Autodesk Fusion 360 part; units mm, degrees
note: some values were not read from the file. Set by a fixed rule: which sketch regions a step uses.
(part 3 of 4)
  spline S86 degree 3 poles (-105.7651, -158.0876) (-108.1851, -156.9591) (-106.086, -147.5724) (-100.1317, -132.8949) knots 0 0 0 0 1 1 1 1
  spline S87 degree 3 poles (-100.1317, -132.8949) (-98.7815, -129.5666) (-97.5292, -125.0086) (-97.3489, -122.7659) knots 0 0 0 0 1 1 1 1
  spline S88 degree 3 poles (-97.3489, -122.7659) (-97.1686, -120.5233) (-96.5325, -118.1966) (-95.9356, -117.5951) knots 0 0 0 0 1 1 1 1
  spline S89 degree 3 poles (-95.9356, -117.5951) (-95.3387, -116.9936) (-94.113, -114.2518) (-93.212, -111.5023) knots 0 0 0 0 1 1 1 1
  spline S90 degree 3 poles (-93.212, -111.5023) (-91.5685, -106.4875) (-88.2032, -100.9795) (-84.6693, -97.5197) knots 0 0 0 0 1 1 1 1
  spline S91 degree 3 poles (-84.6693, -97.5197) (-83.6282, -96.5006) (-82.5684, -95.831) (-82.3142, -96.0317) knots 0 0 0 0 1 1 1 1
  spline S92 degree 3 poles (-82.3142, -96.0317) (-80.8591, -97.1801) (-81.4531, -105.6318) (-83.0888, -107.0535) knots 0 0 0 0 1 1 1 1
  spline S93 degree 3 poles (-83.0888, -107.0535) (-83.9086, -107.766) (-83.3399, -110.3472) (-82.4356, -110.0181) knots 0 0 0 0 1 1 1 1
  spline S94 degree 3 poles (-82.4356, -110.0181) (-81.5449, -109.6939) (-77.0276, -113.218) (-76.5096, -114.6411) knots 0 0 0 0 1 1 1 1
  spline S95 degree 3 poles (-76.5096, -114.6411) (-76.1157, -115.7233) (-75.6688, -115.8539) (-74.1947, -115.3174) knots 0 0 0 0 1 1 1 1
  spline S96 degree 3 poles (-74.1947, -115.3174) (-73.0292, -114.8932) (-71.9308, -114.9941) (-71.1607, -115.5962) knots 0 0 0 0 1 1 1 1
  spline S97 degree 3 poles (-71.1607, -115.5962) (-70.4967, -116.1152) (-69.7314, -116.4591) (-69.4601, -116.3603) knots 0 0 0 0 1 1 1 1
  spline S98 degree 3 poles (-69.4601, -116.3603) (-69.1888, -116.2616) (-67.7713, -116.3006) (-66.31, -116.4471) knots 0 0 0 0 1 1 1 1
  spline S99 degree 3 poles (-66.31, -116.4471) (-58.7633, -116.1747) (-54.7735, -110.4959) (-53.9972, -105.1142) knots 0 0 0 0 1 1 1 1
  spline S100 degree 3 poles (-53.9972, -105.1142) (-53.3719, -100.2884) (-56.959, -94.4448) (-60.8927, -93.8814) knots 0 0 0 0 1 1 1 1
  spline S101 degree 3 poles (-60.8927, -93.8814) (-63.6579, -93.4851) (-63.887, -92.6055) (-62.4815, -87.7805) knots 0 0 0 0 1 1 1 1
  spline S102 degree 3 poles (-62.4815, -87.7805) (-60.4144, -80.6836) (-58.6819, -56.2234) (-59.8595, -50.7648) knots 0 0 0 0 1 1 1 1
  spline S103 degree 3 poles (-59.8595, -50.7648) (-60.45, -48.0282) (-60.4959, -47.9901) (-66.1098, -45.5661) knots 0 0 0 0 1 1 1 1
  spline S104 degree 3 poles (-66.1098, -45.5661) (-72.7999, -42.6775) (-79.68, -40.6969) (-84.3741, -40.3079) knots 0 0 0 0 1 1 1 1
  spline S105 degree 3 poles (-84.3741, -40.3079) (-87.8752, -40.018) (-88.8355, -39.1456) (-87.7319, -37.2577) knots 0 0 0 0 1 1 1 1
  spline S106 degree 3 poles (-87.7319, -37.2577) (-87.3803, -36.6562) (-87.2231, -35.8055) (-87.3826, -35.3672) knots 0 0 0 0 1 1 1 1
  spline S107 degree 3 poles (-87.3826, -35.3672) (-87.8899, -33.9734) (-86.4389, -25.012) (-85.4231, -23.2654) knots 0 0 0 0 1 1 1 1
  spline S108 degree 3 poles (-85.4231, -23.2654) (-84.2448, -21.2393) (-84.8036, -21.3276) (-87.2116, -23.5478) knots 0 0 0 0 1 1 1 1
  spline S109 degree 3 poles (-87.2116, -23.5478) (-88.988, -25.1857) (-89.0133, -25.1867) (-89.5753, -23.6426) knots 0 0 0 0 1 1 1 1
  spline S110 degree 3 poles (-89.5753, -23.6426) (-91.0986, -20.9242) (-96.5777, -20.042) (-99.4834, -22.2152) knots 0 0 0 0 1 1 1 1
  spline S111 degree 3 poles (-99.4834, -22.2152) (-102.7671, -24.1219) (-105.1902, -27.5695) (-103.4783, -30.4373) knots 0 0 0 0 1 1 1 1
  spline S112 degree 3 poles (-103.4783, -30.4373) (-102.821, -31.518) (-102.6423, -32.3115) (-103.0249, -32.4507) knots 0 0 0 0 1 1 1 1
  spline S113 degree 3 poles (-103.0249, -32.4507) (-103.3722, -32.5771) (-103.4148, -32.8712) (-103.1195, -33.1042) knots 0 0 0 0 1 1 1 1
  spline S114 degree 3 poles (-103.1195, -33.1042) (-102.17, -33.8536) (-103.886, -34.7192) (-105.7404, -34.4262) knots 0 0 0 0 1 1 1 1
  spline S115 degree 3 poles (-105.7404, -34.4262) (-106.729, -34.2701) (-107.319, -34.0516) (-107.0516, -33.9408) knots 0 0 0 0 1 1 1 1
  spline S116 degree 3 poles (-107.0516, -33.9408) (-106.7842, -33.83) (-106.9049, -33.4739) (-107.3197, -33.1494) knots 0 0 0 0 1 1 1 1
  spline S117 degree 3 poles (-107.3197, -33.1494) (-108.6187, -32.1334) (-109.3089, -30.4554) (-108.3458, -30.6552) knots 0 0 0 0 1 1 1 1
  spline S118 degree 3 poles (-108.3458, -30.6552) (-107.7548, -30.7777) (-107.7164, -30.5518) (-108.2282, -29.9629) knots 0 0 0 0 1 1 1 1
  spline S119 degree 3 poles (-108.2282, -29.9629) (-108.6756, -29.448) (-108.6885, -28.9597) (-108.2594, -28.7749) knots 0 0 0 0 1 1 1 1
  spline S120 degree 3 poles (-108.2594, -28.7749) (-107.8588, -28.6023) (-108.1586, -28.4465) (-108.9258, -28.4287) knots 0 0 0 0 1 1 1 1
  spline S121 degree 3 poles (-108.9258, -28.4287) (-110.0298, -28.403) (-110.4149, -28.866) (-110.7717, -30.6482) knots 0 0 0 0 1 1 1 1
  spline S122 degree 3 poles (-110.7717, -30.6482) (-111.1259, -32.417) (-111.4051, -32.7562) (-112.0728, -32.2292) knots 0 0 0 0 1 1 1 1
  spline S123 degree 3 poles (-112.0728, -32.2292) (-112.5404, -31.8601) (-113.2203, -31.6275) (-113.5837, -31.7122) knots 0 0 0 0 1 1 1 1
  spline S124 degree 3 poles (-113.5837, -31.7122) (-114.8758, -31.1202) (-118.9006, -30.5) (-119.4232, -30.4738) knots 0 0 0 0 1 1 1 1
  spline S125 degree 3 poles (-119.4232, -30.4738) (-125.5719, -30.4722) (-132.2129, -34.4961) (-136.2209, -38.6484) knots 0 0 0 0 1 1 1 1
  spline S126 degree 3 poles (-136.2209, -38.6484) (-139.7578, -43.5067) (-144.003, -49.2146) (-147.0742, -52.9444) knots 0 0 0 0 1 1 1 1
  spline S127 degree 3 poles (-147.0742, -52.9444) (-148.0276, -54.2206) (-148.1757, -54.2339) (-148.9598, -53.1145) knots 0 0 0 0 1 1 1 1
  spline S128 degree 3 poles (-148.9598, -53.1145) (-150.8779, -46.6854) (-153.7349, -39.6687) (-154.7919, -33.624) knots 0 0 0 0 1 1 1 1
  spline S129 degree 3 poles (-154.7919, -33.624) (-155.1377, -31.5295) (-154.9908, -31.2048) (-153.5956, -30.9793) knots 0 0 0 0 1 1 1 1
  spline S130 degree 3 poles (-153.5956, -30.9793) (-152.7208, -30.838) (-152.0912, -30.4856) (-152.1965, -30.1964) knots 0 0 0 0 1 1 1 1
  spline S131 degree 3 poles (-152.1965, -30.1964) (-152.6058, -29.0718) (-152.5865, -28.6889) (-152.0887, -28.0582) knots 0 0 0 0 1 1 1 1
  spline S132 degree 3 poles (-152.0887, -28.0582) (-151.7288, -27.6023) (-151.9309, -27.195) (-152.7563, -26.7125) knots 0 0 0 0 1 1 1 1
  spline S133 degree 3 poles (-152.7563, -26.7125) (-153.7036, -26.1588) (-153.9953, -26.2199) (-154.2165, -27.0184) knots 0 0 0 0 1 1 1 1
  spline S134 degree 3 poles (-154.2165, -27.0184) (-154.4007, -27.683) (-154.551, -27.4601) (-154.6666, -26.3504) knots 0 0 0 0 1 1 1 1
  spline S135 degree 3 poles (-154.6666, -26.3504) (-155.4003, -19.3112) (-156.3482, -18.6133) (-162.7786, -20.375) knots 0 0 0 0 1 1 1 1
  spline S136 degree 3 poles (-162.7786, -20.375) (-166.2731, -21.3325) (-168.0229, -21.4708) (-169.6944, -20.9217) knots 0 0 0 0 1 1 1 1
  spline S137 degree 3 poles (-169.6944, -20.9217) (-170.9251, -20.5173) (-172.5768, -20.4211) (-173.3647, -20.7079) knots 0 0 0 0 1 1 1 1
  spline S138 degree 3 poles (-173.3647, -20.7079) (-174.7646, -21.2174) (-175.2692, -20.8019) (-177.1846, -17.5625) knots 0 0 0 0 1 1 1 1
  spline S139 degree 3 poles (-177.1846, -17.5625) (-177.5438, -16.9549) (-178.0397, -15.9683) (-178.2865, -15.3701) knots 0 0 0 0 1 1 1 1
  spline S140 degree 3 poles (-178.2865, -15.3701) (-178.5334, -14.7718) (-178.926, -14.524) (-179.1592, -14.8194) knots 0 0 0 0 1 1 1 1
  spline S141 degree 3 poles (-179.1592, -14.8194) (-179.6701, -15.4667) (-181.8024, -11.7834) (-183.7113, -6.9562) knots 0 0 0 0 1 1 1 1
  spline S142 degree 3 poles (-183.7113, -6.9562) (-184.7798, -4.2542) (-185.4511, -3.3311) (-186.5872, -3.0015) knots 0 0 0 0 1 1 1 1
  spline S143 degree 3 poles (-186.5872, -3.0015) (-187.4809, -2.7423) (-188.3354, -1.8401) (-188.7399, -0.7287) knots 0 0 0 0 1 1 1 1
  line L100 (-188.7399, -0.7287) -> (-189.0051, 0)
  line L101 (-189.0051, 0) -> (-213.5849, 0)
  line L102 (-213.5849, 0) -> (-217.2124, -1.9134)
  spline S144 degree 3 poles (-217.2124, -1.9134) (-227.6497, -7.419) (-230.8144, -9.6389) (-238.2871, -16.6962) knots -1 -1 -1 -1 0 0 0 0
  spline S145 degree 3 poles (-238.2871, -16.6962) (-241.2992, -19.5409) (-242.2366, -21.2822) (-241.7525, -23.1333) knots -1 -1 -1 -1 0 0 0 0
  spline S146 degree 3 poles (-241.7525, -23.1333) (-241.1428, -25.4651) (-244.6533, -29.9662) (-247.1739, -30.0848) knots -1 -1 -1 -1 0 0 0 0
  spline S147 degree 3 poles (-247.1739, -30.0848) (-249.0728, -30.1745) (-269.6477, -43.1315) (-278.0022, -49.4997) knots -1 -1 -1 -1 0 0 0 0
  spline S148 degree 3 poles (-278.0022, -49.4997) (-282.9288, -53.2546) (-290.5449, -59.0168) (-294.9276, -62.3044) knots -1 -1 -1 -1 0 0 0 0
  line L103 (-294.9276, -62.3044) -> (-302.8961, -68.2819)
  line L104 (-302.8961, -68.2819) -> (-303.532, -63.8424)
  spline S149 degree 3 poles (-303.532, -63.8424) (-303.8818, -61.4006) (-304.0603, -58.0584) (-303.9287, -56.4153) knots -1 -1 -1 -1 0 0 0 0
  spline S150 degree 3 poles (-303.9287, -56.4153) (-303.7162, -53.761) (-304.1228, -53.4473) (-307.5734, -53.6039) knots -1 -1 -1 -1 0 0 0 0
  spline S151 degree 3 poles (-307.5734, -53.6039) (-309.7095, -53.7008) (-311.4572, -53.2657) (-311.4572, -52.6371) knots -1 -1 -1 -1 0 0 0 0
  spline S152 degree 3 poles (-311.4572, -52.6371) (-311.4572, -52.0085) (-312.0037, -51.8319) (-312.6717, -52.2447) knots -1 -1 -1 -1 0 0 0 0
  spline S153 degree 3 poles (-312.6717, -52.2447) (-313.3397, -52.6576) (-313.5769, -53.4959) (-313.1987, -54.1078) knots -1 -1 -1 -1 0 0 0 0
  spline S154 degree 3 poles (-313.1987, -54.1078) (-312.8205, -54.7196) (-313.0432, -55.2202) (-313.6936, -55.2202) knots -1 -1 -1 -1 0 0 0 0
  spline S155 degree 3 poles (-313.6936, -55.2202) (-314.344, -55.2202) (-315.0479, -54.0652) (-315.2579, -52.6535) knots -1 -1 -1 -1 0 0 0 0
  spline S156 degree 3 poles (-315.2579, -52.6535) (-315.9974, -47.6815) (-318.8808, -47.3363) (-329.5358, -50.9442) knots -1 -1 -1 -1 0 0 0 0
  spline S157 degree 3 poles (-329.5358, -50.9442) (-334.9861, -52.7898) (-340.6591, -55.095) (-342.1423, -56.0668) knots -1 -1 -1 -1 0 0 0 0
  spline S158 degree 3 poles (-342.1423, -56.0668) (-344.0393, -57.3097) (-346.2683, -57.5922) (-349.6584, -57.0194) knots -1 -1 -1 -1 0 0 0 0
  spline S159 degree 3 poles (-349.6584, -57.0194) (-352.3092, -56.5716) (-354.4815, -55.8492) (-354.4861, -55.414) knots -1 -1 -1 -1 0 0 0 0
  spline S160 degree 3 poles (-354.4861, -55.414) (-354.4925, -54.769) (-356.973, -52.9332) (-363.8641, -48.4729) knots -1 -1 -1 -1 0 0 0 0
  spline S161 degree 3 poles (-363.8641, -48.4729) (-364.097, -48.3222) (-362.0803, -44.2) (-359.3827, -39.3133) knots -1 -1 -1 -1 0 0 0 0
  spline S162 degree 3 poles (-359.3827, -39.3133) (-356.685, -34.4266) (-354.4778, -29.5947) (-354.4778, -28.5764) knots -1 -1 -1 -1 0 0 0 0
  spline S163 degree 3 poles (-354.4778, -28.5764) (-354.4778, -27.5581) (-351.6792, -21.4404) (-348.2586, -14.9809) knots -1 -1 -1 -1 0 0 0 0
  spline S164 degree 3 poles (-348.2586, -14.9809) (-345.7092, -10.1666) (-342.6343, -4.2707) (-340.44, 0) knots -1 -1 -1 -1 -0.254706 -0.254706 -0.254706 -0.254706
  line L105 (-340.44, 0) -> (-355.8194, 0)
  spline S165 degree 3 poles (-355.8194, 0) (-360.8369, -5.9766) (-365.8588, -13.4774) (-366.89, -16.9696) knots -0.735419 -0.735419 -0.735419 -0.735419 0 0 0 0
  spline S166 degree 3 poles (-366.89, -16.9696) (-368.1026, -21.0773) (-379.0998, -35.0894) (-384.1975, -39.0223) knots -1 -1 -1 -1 0 0 0 0
  spline S167 degree 3 poles (-384.1975, -39.0223) (-389.0192, -42.7421) (-392.428, -47.1455) (-393.8711, -51.5183) knots -1 -1 -1 -1 0 0 0 0
  spline S168 degree 3 poles (-393.8711, -51.5183) (-394.7608, -54.2141) (-395.926, -56.4196) (-396.4605, -56.4196) knots -1 -1 -1 -1 0 0 0 0
  spline S169 degree 3 poles (-396.4605, -56.4196) (-396.995, -56.4196) (-399.8352, -55.2522) (-402.7721, -53.8254) knots -1 -1 -1 -1 0 0 0 0
  spline S170 degree 3 poles (-402.7721, -53.8254) (-407.2094, -51.6696) (-408.4269, -51.4923) (-409.9744, -52.7766) knots -1 -1 -1 -1 0 0 0 0
  spline S171 degree 3 poles (-409.9744, -52.7766) (-412.2152, -54.6361) (-412.3844, -57.7837) (-410.3529, -59.8152) knots -1 -1 -1 -1 0 0 0 0
  spline S172 degree 3 poles (-410.3529, -59.8152) (-409.1713, -60.9969) (-409.1757, -61.4884) (-410.3748, -62.2295) knots -1 -1 -1 -1 0 0 0 0
  spline S173 degree 3 poles (-410.3748, -62.2295) (-413.7834, -64.3357) (-414.078, -70.2597) (-411.269, -80.2141) knots -1 -1 -1 -1 0 0 0 0
  spline S174 degree 3 poles (-411.269, -80.2141) (-409.7681, -85.5329) (-407.9951, -90.5559) (-407.329, -91.376) knots -1 -1 -1 -1 0 0 0 0
  spline S175 degree 3 poles (-407.329, -91.376) (-406.6629, -92.1961) (-405.899, -100.3959) (-405.6314, -109.5978) knots -1 -1 -1 -1 0 0 0 0
  spline S176 degree 3 poles (-405.6314, -109.5978) (-405.2611, -122.3336) (-404.6599, -127.2412) (-403.1133, -130.1526) knots -1 -1 -1 -1 0 0 0 0
  spline S177 degree 3 poles (-403.1133, -130.1526) (-401.9958, -132.2563) (-401.0815, -135.2288) (-401.0815, -136.7584) knots -1 -1 -1 -1 0 0 0 0
  spline S178 degree 3 poles (-401.0815, -136.7584) (-401.0815, -138.2879) (-400.2443, -140.7345) (-399.2212, -142.1953) knots -1 -1 -1 -1 0 0 0 0
  spline S179 degree 3 poles (-399.2212, -142.1953) (-397.754, -144.2899) (-397.6998, -144.8513) (-398.9647, -144.8513) knots -1 -1 -1 -1 0 0 0 0
  spline S180 degree 3 poles (-398.9647, -144.8513) (-399.8472, -144.8513) (-403.7766, -148.2524) (-407.6974, -152.4097) knots -1 -1 -1 -1 0 0 0 0
  spline S181 degree 3 poles (-407.6974, -152.4097) (-412.4596, -157.459) (-416.0694, -160.217) (-418.5714, -160.7174) knots -1 -1 -1 -1 0 0 0 0
  spline S182 degree 3 poles (-418.5714, -160.7174) (-423.3796, -161.6792) (-430.8685, -166.7624) (-433.5752, -170.9019) knots -1 -1 -1 -1 0 0 0 0
  spline S183 degree 3 poles (-433.5752, -170.9019) (-438.1872, -177.9547) (-449.9333, -190.6228) (-454.8506, -193.8468) knots -1 -1 -1 -1 0 0 0 0
  spline S184 degree 3 poles (-454.8506, -193.8468) (-456.9343, -195.2125) (-460.9906, -198.8048) (-469.9, -207.2338) knots -1 -1 -1 -1 -0.162411 -0.162411 -0.162411 -0.162411
  line L106 (-469.9, -207.2338) -> (-469.9, -215.9)
  line L107 (-469.9, -215.9) -> (-76.8192, -215.9)
  line L108 (-133.35, -107.95) -> (-154.94, -107.95)
  circle A87 centre (-154.94, -107.95) radius 3.175
  circle A88 centre (-154.94, -107.95) radius 6.35
  dimension "d72" = 6.35
  dimension "d89" = 12.7
  constraint horizontal L108
  constraint coincident L108.end A87.centre
  measures "d72" diameter of A87
  measures "d89" diameter of A88
extrude "Extrude3" cut sketch "Sketch3" against normal blind 508 contours A87 bodies 1
extrude "Extrude4" add sketch "Sketch1" along normal blind 25.4 contours A91 bodies 1
extrude "Extrude5" cut 1 faces at (207.9539, 60.1803, 38.1) along direction (0, 0, -1) blind 12.7 on bodies 1 bodies 1
extrude "Extrude6" add sketch "Sketch1" along normal blind 25.4 contours A2 | L8 L13 L17 L23 L24 L28 A9 A10 A11 A12 A13 A14 | L9 L12 L19 L21 L26 L36 A15 A16 A17 A18 A19 A20 | L10 L14 L16 L18 L20 L22 A3 A4 A5 A6 A7 A8 | L11 L15 L25 L27 L29 L37 A21 A22 A23 A24 A25 A26 | L38 L41 L45 L47 A30 A34 A36 A40 L57 A42 A43 L59 | L39 L44 A27 A29 L50 L53 A35 A38 A39 A41 L58 L60 A87 | L40 L46 L48 A28 L51 L52 A31 A32 A33 L55 A37 A44 | L62 L65 L67 A47 A51 L80 L82 A58 A59 L88 A83 A86 | A45 L75 A60 L101 L102 L104 A70 L108 A74 L115 A78 A80 | L63 L64 L68 A46 L73 A48 A50 A52 A56 L87 A61 L91 | L66 L69 L70 A49 A53 A54 A55 L81 A57 L83 L86 A82 L121 | L71 A63 L98 L100 A68 A71 A72 L109 L113 A76 L114 A77 | L72 A62 A65 L94 L96 A66 L99 A67 L110 A73 L111 A75 | L79 A64 L92 L93 L103 A69 L107 L112 A79 A81 A84 A85 L122 | A98 | A102 bodies 1
extrude "Extrude7" add sketch "Sketch3" against normal blind 38.1 contours A87 bodies 1
extrude "Extrude8" cut sketch "Sketch3" against normal blind 12.7 contours A87 bodies 1
extrude "Extrude9" add sketch "Sketch1" along normal blind 25.4 contours L39 A87 picked at (189.8635, 111.434) bodies 1
extrude "Extrude10" cut sketch "Sketch1" along normal blind 508 contours A2 | L8 L13 L17 L23 L24 L28 A9 A10 A11 A12 A13 A14 | L9 L12 L19 L21 L26 L36 A15 A16 A17 A18 A19 A20 | L10 L14 L16 L18 L20 L22 A3 A4 A5 A6 A7 A8 | L11 L15 L25 L27 L29 L37 A21 A22 A23 A24 A25 A26 | L38 L41 L45 L47 A30 A34 A36 A40 L57 A42 A43 L59 | L39 L44 A27 A29 L50 L53 A35 A38 A39 A41 L58 L60 A87 | L39 A87 | L39 A87 | L40 L46 L48 A28 L51 L52 A31 A32 A33 L55 A37 A44 | L62 L65 L67 A47 A51 L80 L82 A58 A59 L88 A83 A86 | A45 L75 A60 L101 L102 L104 A70 L108 A74 L115 A78 A80 | L63 L64 L68 A46 L73 A48 A50 A52 A56 L87 A61 L91 | L66 L69 L70 A49 A53 A54 A55 L81 A57 L83 L86 A82 L121 | L71 A63 L98 L100 A68 A71 A72 L109 L113 A76 L114 A77 | L72 A62 A65 L94 L96 A66 L99 A67 L110 A73 L111 A75 | L79 A64 L92 L93 L103 A69 L107 L112 A79 A81 A84 A85 L122 | L116 L117 L118 L119 L120 L125 | A88 | A89 | A90 | A93 | A94 | A95 | A96 | A98 | A102 bodies 1
extrude "Extrude11" cut sketch "Sketch3" against normal blind 254 contours A87 | A88 bodies 1
extrude "Extrude12" add sketch "Sketch1" along normal blind 25.4 contours A93 | A94 | A95 | A96 bodies 1
extrude "Extrude13" add sketch "Sketch3" against normal blind 38.1 contours A88 bodies 1
extrude "Extrude14" cut sketch "Sketch3" against normal blind 12.7 contours A88 bodies 1
extrude "Extrude15" add sketch "Sketch1" along normal blind 25.4 contours L39 A87 | L116 L117 L118 L119 L120 L125 | A88 | A89 | A90 picked at (189.0956, 109.9792) bodies 1
extrude "Extrude16" cut sketch "Sketch1" along normal blind 508 contours A93 | A94 | A95 | A96 bodies 1
sketch "Sketch9" plane through (0, 0, 0) normal (0, 0, 1) x (1, 0, 0)
  line L0 (298.45, 190.5) -> (298.45, 101.6)
  line L1 (171.45, 101.6) -> (171.45, 190.5)
  line L2 (298.45, 146.05) -> (171.45, 146.05)
  line L3 (297.18, 189.23) -> (172.72, 189.23)
  line L4 (172.72, 189.23) -> (172.72, 102.87)
  line L5 (172.72, 102.87) -> (297.18, 102.87)
  line L6 (297.18, 102.87) -> (297.18, 189.23)
  line L7 (297.18, 189.23) -> (172.72, 102.87) construction
  line L8 (172.72, 189.23) -> (297.18, 102.87) construction
  point P0 (234.95, 146.05)
  dimension "d102" = 124.46
  dimension "d103" = 86.36
  constraint midpoint L0 L2.start
  constraint midpoint L1 L2.end
  constraint horizontal L3
  constraint perpendicular L3 L4
  constraint parallel L3 L5
  constraint parallel L4 L6
  constraint coincident L7 P0
  constraint coincident L8 P0
  constraint midpoint L2 P0
  measures "d102" distance of L4.end L5.end
  measures "d103" distance of L3.end L4.end
extrude "Extrude17" cut sketch "Sketch1" along normal blind 254 contours L0 L1 L3 L4 L5 L6 L7 | L1 L2 L3 L6 L123 L124 bodies 1 makes body 2 at (135.9617, 113.7381, 16.9333)
extrude "Extrude18" cut 1 faces at (135.3022, 107.6345, 0) along direction (0, 0, 1) blind 254 on bodies 2 bodies 2
sketch "Sketch10" plane through (0, 0, 25.4) normal (0, 0, 1) x (-1, 0, 0)
  arc A0 (-196.478, -134.992) -> (-197.3761, -134.62) centre (-197.3761, -135.89) ccw
  line L0 (-196.478, -134.992) -> (-193.938, -137.532)
  arc A1 (-193.938, -139.328) -> (-193.938, -137.532) centre (-194.8361, -138.43) ccw
  line L1 (-193.938, -139.328) -> (-196.478, -141.868)
  arc A2 (-197.3761, -142.24) -> (-196.478, -141.868) centre (-197.3761, -140.97) ccw
  line L2 (-197.3761, -142.24) -> (-214.104, -142.24)
  arc A3 (-215.002, -141.868) -> (-214.104, -142.24) centre (-214.104, -140.97) ccw
  line L3 (-215.002, -141.868) -> (-217.542, -139.328)
  arc A4 (-217.542, -137.532) -> (-217.542, -139.328) centre (-216.644, -138.43) ccw
  line L4 (-217.542, -137.532) -> (-215.002, -134.992)
  arc A5 (-214.104, -134.62) -> (-215.002, -134.992) centre (-214.104, -135.89) ccw
  line L5 (-214.104, -134.62) -> (-197.3761, -134.62)
  arc A6 (-215.002, -172.348) -> (-214.104, -172.72) centre (-214.104, -171.45) ccw
  line L6 (-215.002, -172.348) -> (-217.542, -169.808)
  arc A7 (-217.542, -168.012) -> (-217.542, -169.808) centre (-216.644, -168.91) ccw
  line L7 (-217.542, -168.012) -> (-215.002, -165.472)
  arc A8 (-214.104, -165.1) -> (-215.002, -165.472) centre (-214.104, -166.37) ccw
  line L8 (-214.104, -165.1) -> (-197.3761, -165.1)
  arc A9 (-196.478, -165.472) -> (-197.3761, -165.1) centre (-197.3761, -166.37) ccw
  line L9 (-196.478, -165.472) -> (-193.938, -168.012)
  arc A10 (-193.938, -169.808) -> (-193.938, -168.012) centre (-194.8361, -168.91) ccw
  line L10 (-193.938, -169.808) -> (-196.478, -172.348)
  arc A11 (-197.3761, -172.72) -> (-196.478, -172.348) centre (-197.3761, -171.45) ccw
  line L11 (-197.3761, -172.72) -> (-214.104, -172.72)
  line L12 (-215.9, -113.5561) -> (-215.9, -132.8239)
  arc A12 (-216.272, -133.7219) -> (-215.9, -132.8239) centre (-217.17, -132.8239) ccw
  line L13 (-216.272, -133.7219) -> (-218.8119, -136.2619)
  arc A13 (-220.608, -136.2619) -> (-218.8119, -136.2619) centre (-219.71, -135.3638) ccw
  line L14 (-220.608, -136.2619) -> (-223.148, -133.7219)
  arc A14 (-223.52, -132.8238) -> (-223.148, -133.7219) centre (-222.25, -132.8238) ccw
  line L15 (-223.52, -132.8238) -> (-223.52, -113.556)
  arc A15 (-223.148, -112.658) -> (-223.52, -113.556) centre (-222.25, -113.556) ccw
  line L16 (-223.148, -112.658) -> (-220.608, -110.118)
  arc A16 (-218.812, -110.118) -> (-220.608, -110.118) centre (-219.71, -111.0161) ccw
  line L17 (-218.812, -110.118) -> (-216.272, -112.658)
  arc A17 (-215.9, -113.5561) -> (-216.272, -112.658) centre (-217.17, -113.5561) ccw
  arc A18 (-253.628, -112.658) -> (-254, -113.5561) centre (-252.73, -113.5561) ccw
  line L18 (-253.628, -112.658) -> (-251.088, -110.118)
  arc A19 (-249.292, -110.118) -> (-251.088, -110.118) centre (-250.19, -111.0161) ccw
  line L19 (-249.292, -110.118) -> (-246.752, -112.658)
  arc A20 (-246.38, -113.556) -> (-246.752, -112.658) centre (-247.65, -113.556) ccw
  line L20 (-246.38, -113.556) -> (-246.38, -132.8238)
  arc A21 (-246.752, -133.7219) -> (-246.38, -132.8238) centre (-247.65, -132.8238) ccw
  line L21 (-246.752, -133.7219) -> (-249.292, -136.2619)
  arc A22 (-251.0881, -136.2619) -> (-249.292, -136.2619) centre (-250.19, -135.3638) ccw
  line L22 (-251.0881, -136.2619) -> (-253.628, -133.7219)
  arc A23 (-254, -132.8239) -> (-253.628, -133.7219) centre (-252.73, -132.8239) ccw
  line L23 (-254, -132.8239) -> (-254, -113.5561)
  arc A24 (-272.5239, -134.62) -> (-273.422, -134.992) centre (-272.5239, -135.89) ccw
  line L24 (-272.5239, -134.62) -> (-255.796, -134.62)
  arc A25 (-254.898, -134.992) -> (-255.796, -134.62) centre (-255.796, -135.89) ccw
  line L25 (-254.898, -134.992) -> (-252.358, -137.532)
  arc A26 (-252.358, -139.328) -> (-252.358, -137.532) centre (-253.256, -138.43) ccw
  line L26 (-252.358, -139.328) -> (-254.898, -141.868)
  arc A27 (-255.796, -142.24) -> (-254.898, -141.868) centre (-255.796, -140.97) ccw
  line L27 (-255.796, -142.24) -> (-272.5239, -142.24)
  arc A28 (-273.422, -141.868) -> (-272.5239, -142.24) centre (-272.5239, -140.97) ccw
  line L28 (-273.422, -141.868) -> (-275.962, -139.328)
  arc A29 (-275.962, -137.532) -> (-275.962, -139.328) centre (-275.0639, -138.43) ccw
  line L29 (-275.962, -137.532) -> (-273.422, -134.992)
  arc A30 (-275.962, -168.012) -> (-275.962, -169.808) centre (-275.0639, -168.91) ccw
  line L30 (-275.962, -168.012) -> (-273.422, -165.472)
  arc A31 (-272.5239, -165.1) -> (-273.422, -165.472) centre (-272.5239, -166.37) ccw
  line L31 (-272.5239, -165.1) -> (-255.796, -165.1)
  arc A32 (-254.898, -165.472) -> (-255.796, -165.1) centre (-255.796, -166.37) ccw
  line L32 (-254.898, -165.472) -> (-252.358, -168.012)
  arc A33 (-252.358, -169.808) -> (-252.358, -168.012) centre (-253.256, -168.91) ccw
  line L33 (-252.358, -169.808) -> (-254.898, -172.348)
  arc A34 (-255.796, -172.72) -> (-254.898, -172.348) centre (-255.796, -171.45) ccw
  line L34 (-255.796, -172.72) -> (-272.5239, -172.72)
  arc A35 (-273.422, -172.348) -> (-272.5239, -172.72) centre (-272.5239, -171.45) ccw
  line L35 (-273.422, -172.348) -> (-275.962, -169.808)
  arc A36 (-279.028, -166.742) -> (-277.232, -166.742) centre (-278.13, -165.844) ccw
  line L36 (-279.028, -166.742) -> (-281.568, -164.202)
  arc A37 (-281.94, -163.3039) -> (-281.568, -164.202) centre (-280.67, -163.3039) ccw
  line L37 (-281.94, -163.3039) -> (-281.94, -144.036)
  arc A38 (-281.568, -143.138) -> (-281.94, -144.036) centre (-280.67, -144.036) ccw
  line L38 (-281.568, -143.138) -> (-279.028, -140.598)
  arc A39 (-277.232, -140.598) -> (-279.028, -140.598) centre (-278.13, -141.496) ccw
  line L39 (-277.232, -140.598) -> (-274.692, -143.138)
  arc A40 (-274.32, -144.036) -> (-274.692, -143.138) centre (-275.59, -144.036) ccw
  line L40 (-274.32, -144.036) -> (-274.32, -163.3039)
  arc A41 (-274.692, -164.202) -> (-274.32, -163.3039) centre (-275.59, -163.3039) ccw
  line L41 (-274.692, -164.202) -> (-277.232, -166.742)
  arc A42 (-190.872, -140.598) -> (-192.668, -140.598) centre (-191.77, -141.496) ccw
  line L42 (-190.872, -140.598) -> (-188.332, -143.138)
  arc A43 (-187.96, -144.036) -> (-188.332, -143.138) centre (-189.23, -144.036) ccw
  line L43 (-187.96, -144.036) -> (-187.96, -163.3039)
  arc A44 (-188.332, -164.202) -> (-187.96, -163.3039) centre (-189.23, -163.3039) ccw
  line L44 (-188.332, -164.202) -> (-190.872, -166.742)
  arc A45 (-192.668, -166.742) -> (-190.872, -166.742) centre (-191.77, -165.844) ccw
  line L45 (-192.668, -166.742) -> (-195.208, -164.202)
  arc A46 (-195.58, -163.3039) -> (-195.208, -164.202) centre (-194.31, -163.3039) ccw
  line L46 (-195.58, -163.3039) -> (-195.58, -144.036)
  arc A47 (-195.208, -143.138) -> (-195.58, -144.036) centre (-194.31, -144.036) ccw
  line L47 (-195.208, -143.138) -> (-192.668, -140.598)
  arc A48 (-253.628, -143.1381) -> (-254, -144.0361) centre (-252.73, -144.0361) ccw
  line L48 (-253.628, -143.1381) -> (-251.0881, -140.5981)
  arc A49 (-249.292, -140.5981) -> (-251.0881, -140.5981) centre (-250.19, -141.4962) ccw
  line L49 (-249.292, -140.5981) -> (-246.752, -143.1381)
  arc A50 (-246.38, -144.0362) -> (-246.752, -143.1381) centre (-247.65, -144.0362) ccw
  line L50 (-246.38, -144.0362) -> (-246.38, -163.304)
  arc A51 (-246.752, -164.202) -> (-246.38, -163.304) centre (-247.65, -163.304) ccw
  line L51 (-246.752, -164.202) -> (-249.292, -166.742)
  arc A52 (-251.088, -166.742) -> (-249.292, -166.742) centre (-250.19, -165.8439) ccw
  line L52 (-251.088, -166.742) -> (-253.628, -164.202)
  arc A53 (-254, -163.3039) -> (-253.628, -164.202) centre (-252.73, -163.3039) ccw
  line L53 (-254, -163.3039) -> (-254, -144.0361)
  arc A54 (-277.232, -110.118) -> (-279.028, -110.118) centre (-278.13, -111.016) ccw
  line L54 (-277.232, -110.118) -> (-274.692, -112.658)
  arc A55 (-274.32, -113.5561) -> (-274.692, -112.658) centre (-275.59, -113.5561) ccw
  line L55 (-274.32, -113.5561) -> (-274.32, -132.824)
  arc A56 (-274.692, -133.722) -> (-274.32, -132.824) centre (-275.59, -132.824) ccw
  line L56 (-274.692, -133.722) -> (-277.232, -136.262)
  arc A57 (-279.028, -136.262) -> (-277.232, -136.262) centre (-278.13, -135.364) ccw
  line L57 (-279.028, -136.262) -> (-281.568, -133.722)
  arc A58 (-281.94, -132.824) -> (-281.568, -133.722) centre (-280.67, -132.824) ccw
  line L58 (-281.94, -132.824) -> (-281.94, -113.5561)
  arc A59 (-281.568, -112.658) -> (-281.94, -113.5561) centre (-280.67, -113.5561) ccw
  line L59 (-281.568, -112.658) -> (-279.028, -110.118)
  arc A60 (-254.898, -104.512) -> (-255.796, -104.14) centre (-255.796, -105.41) ccw
  line L60 (-254.898, -104.512) -> (-252.358, -107.052)
  arc A61 (-252.358, -108.848) -> (-252.358, -107.052) centre (-253.256, -107.95) ccw
  line L61 (-252.358, -108.848) -> (-254.898, -111.388)
  arc A62 (-255.796, -111.76) -> (-254.898, -111.388) centre (-255.796, -110.49) ccw
  line L62 (-255.796, -111.76) -> (-272.5239, -111.76)
  arc A63 (-273.422, -111.388) -> (-272.5239, -111.76) centre (-272.5239, -110.49) ccw
  line L63 (-273.422, -111.388) -> (-275.962, -108.848)
  arc A64 (-275.962, -107.052) -> (-275.962, -108.848) centre (-275.0639, -107.95) ccw
  line L64 (-275.962, -107.052) -> (-273.422, -104.512)
  arc A65 (-272.5239, -104.14) -> (-273.422, -104.512) centre (-272.5239, -105.41) ccw
  line L65 (-272.5239, -104.14) -> (-255.796, -104.14)
  arc A66 (-223.52, -163.304) -> (-223.148, -164.202) centre (-222.25, -163.304) ccw
  line L66 (-223.52, -163.304) -> (-223.52, -144.0362)
  arc A67 (-223.148, -143.1381) -> (-223.52, -144.0362) centre (-222.25, -144.0362) ccw
  line L67 (-223.148, -143.1381) -> (-220.608, -140.5981)
  arc A68 (-218.8119, -140.5981) -> (-220.608, -140.5981) centre (-219.71, -141.4962) ccw
  line L68 (-218.8119, -140.5981) -> (-216.272, -143.1381)
  arc A69 (-215.9, -144.0361) -> (-216.272, -143.1381) centre (-217.17, -144.0361) ccw
  line L69 (-215.9, -144.0361) -> (-215.9, -163.3039)
  arc A70 (-216.272, -164.202) -> (-215.9, -163.3039) centre (-217.17, -163.3039) ccw
  line L70 (-216.272, -164.202) -> (-218.812, -166.742)
  arc A71 (-220.608, -166.742) -> (-218.812, -166.742) centre (-219.71, -165.8439) ccw
  line L71 (-220.608, -166.742) -> (-223.148, -164.202)
  arc A72 (-214.104, -104.14) -> (-215.002, -104.512) centre (-214.104, -105.41) ccw
  line L72 (-214.104, -104.14) -> (-197.3761, -104.14)
  arc A73 (-196.478, -104.512) -> (-197.3761, -104.14) centre (-197.3761, -105.41) ccw
  line L73 (-196.478, -104.512) -> (-193.938, -107.052)
  arc A74 (-193.938, -108.848) -> (-193.938, -107.052) centre (-194.8361, -107.95) ccw
  line L74 (-193.938, -108.848) -> (-196.478, -111.388)
  arc A75 (-197.3761, -111.76) -> (-196.478, -111.388) centre (-197.3761, -110.49) ccw
  line L75 (-197.3761, -111.76) -> (-214.104, -111.76)
  arc A76 (-215.002, -111.388) -> (-214.104, -111.76) centre (-214.104, -110.49) ccw
  line L76 (-215.002, -111.388) -> (-217.542, -108.848)
  arc A77 (-217.542, -107.052) -> (-217.542, -108.848) centre (-216.644, -107.95) ccw
  line L77 (-217.542, -107.052) -> (-215.002, -104.512)
  arc A78 (-190.872, -110.118) -> (-192.668, -110.118) centre (-191.77, -111.016) ccw
  line L78 (-190.872, -110.118) -> (-188.332, -112.658)
  arc A79 (-187.96, -113.5561) -> (-188.332, -112.658) centre (-189.23, -113.5561) ccw
  line L79 (-187.96, -113.5561) -> (-187.96, -132.824)
  arc A80 (-188.332, -133.722) -> (-187.96, -132.824) centre (-189.23, -132.824) ccw
  line L80 (-188.332, -133.722) -> (-190.872, -136.262)
  arc A81 (-192.668, -136.262) -> (-190.872, -136.262) centre (-191.77, -135.364) ccw
  line L81 (-192.668, -136.262) -> (-195.208, -133.722)
  arc A82 (-195.58, -132.824) -> (-195.208, -133.722) centre (-194.31, -132.824) ccw
  line L82 (-195.58, -132.824) -> (-195.58, -113.5561)
  arc A83 (-195.208, -112.658) -> (-195.58, -113.5561) centre (-194.31, -113.5561) ccw
  line L83 (-195.208, -112.658) -> (-192.668, -110.118)
  circle A84 centre (-234.95, -107.95) radius 3.175
  line L84 (-171.45, -101.6) -> (-298.45, -101.6)
  line L85 (-298.45, -101.6) -> (-298.45, -190.5)
  line L86 (-298.45, -190.5) -> (-171.45, -190.5)
  line L87 (-171.45, -190.5) -> (-171.45, -101.6)
  line L88 (-297.18, -189.23) -> (-172.72, -189.23)
  line L89 (-172.72, -189.23) -> (-172.72, -102.87)
  line L90 (-172.72, -102.87) -> (-297.18, -102.87)
  line L91 (-297.18, -102.87) -> (-297.18, -189.23)
  line L92 (-297.18, -189.23) -> (-172.72, -102.87) construction
  line L93 (-172.72, -189.23) -> (-297.18, -102.87) construction
  point P0 (-234.95, -146.05)
  dimension "d108" = 124.46
  dimension "d109" = 86.36
  constraint horizontal L88
  constraint perpendicular L88 L89
  constraint parallel L88 L90
  constraint parallel L89 L91
  constraint coincident L92 P0
  constraint coincident L93 P0
  measures "d108" distance of L89.end L90.end
  measures "d109" distance of L88.end L89.end
extrude "Extrude19" cut sketch "Sketch10" against normal blind 254 contours L84 L85 L86 L87 bodies 1
extrude "Extrude20" cut 1 faces at (228.0013, 183.7267, 25.4) along direction (0, 0, -1) blind 6.35 on bodies 1 bodies 1
sketch "Sketch11" plane through (0, 0, 0) normal (0, 0, -1) x (1, 0, 0)
  line L0 (297.18, -102.87) -> (172.72, -102.87)
  line L1 (172.72, -102.87) -> (172.72, -189.23)
  line L2 (172.72, -189.23) -> (297.18, -189.23)
  line L3 (297.18, -189.23) -> (297.18, -102.87)
  arc A0 (197.3761, -134.62) -> (196.478, -134.992) centre (197.3761, -135.89) ccw
  line L4 (197.3761, -134.62) -> (214.104, -134.62)
  arc A1 (215.002, -134.992) -> (214.104, -134.62) centre (214.104, -135.89) ccw
  line L5 (215.002, -134.992) -> (217.542, -137.532)
  arc A2 (217.542, -139.328) -> (217.542, -137.532) centre (216.644, -138.43) ccw
  line L6 (217.542, -139.328) -> (215.002, -141.868)
  arc A3 (214.104, -142.24) -> (215.002, -141.868) centre (214.104, -140.97) ccw
  line L7 (214.104, -142.24) -> (197.3761, -142.24)
  arc A4 (196.478, -141.868) -> (197.3761, -142.24) centre (197.3761, -140.97) ccw
  line L8 (196.478, -141.868) -> (193.938, -139.328)
  arc A5 (193.938, -137.532) -> (193.938, -139.328) centre (194.8361, -138.43) ccw
  line L9 (193.938, -137.532) -> (196.478, -134.992)
  arc A6 (214.104, -172.72) -> (215.002, -172.348) centre (214.104, -171.45) ccw
  line L10 (214.104, -172.72) -> (197.3761, -172.72)
  arc A7 (196.478, -172.348) -> (197.3761, -172.72) centre (197.3761, -171.45) ccw
  line L11 (196.478, -172.348) -> (193.938, -169.808)
  arc A8 (193.938, -168.012) -> (193.938, -169.808) centre (194.8361, -168.91) ccw
  line L12 (193.938, -168.012) -> (196.478, -165.472)
  arc A9 (197.3761, -165.1) -> (196.478, -165.472) centre (197.3761, -166.37) ccw
  line L13 (197.3761, -165.1) -> (214.104, -165.1)
  arc A10 (215.002, -165.472) -> (214.104, -165.1) centre (214.104, -166.37) ccw
  line L14 (215.002, -165.472) -> (217.542, -168.012)
  arc A11 (217.542, -169.808) -> (217.542, -168.012) centre (216.644, -168.91) ccw
  line L15 (217.542, -169.808) -> (215.002, -172.348)
  line L16 (215.9, -132.8239) -> (215.9, -113.5561)
  arc A12 (216.272, -112.658) -> (215.9, -113.5561) centre (217.17, -113.5561) ccw
  line L17 (216.272, -112.658) -> (218.812, -110.118)
  arc A13 (220.608, -110.118) -> (218.812, -110.118) centre (219.71, -111.0161) ccw
  line L18 (220.608, -110.118) -> (223.148, -112.658)
  arc A14 (223.52, -113.556) -> (223.148, -112.658) centre (222.25, -113.556) ccw
  line L19 (223.52, -113.556) -> (223.52, -132.8238)
  arc A15 (223.148, -133.7219) -> (223.52, -132.8238) centre (222.25, -132.8238) ccw
  line L20 (223.148, -133.7219) -> (220.608, -136.2619)
  arc A16 (218.8119, -136.2619) -> (220.608, -136.2619) centre (219.71, -135.3638) ccw
  line L21 (218.8119, -136.2619) -> (216.272, -133.7219)
  arc A17 (215.9, -132.8239) -> (216.272, -133.7219) centre (217.17, -132.8239) ccw
  arc A18 (254, -113.5561) -> (253.628, -112.658) centre (252.73, -113.5561) ccw
  line L22 (254, -113.5561) -> (254, -132.8239)
  arc A19 (253.628, -133.7219) -> (254, -132.8239) centre (252.73, -132.8239) ccw
  line L23 (253.628, -133.7219) -> (251.0881, -136.2619)
  arc A20 (249.292, -136.2619) -> (251.0881, -136.2619) centre (250.19, -135.3638) ccw
  line L24 (249.292, -136.2619) -> (246.752, -133.7219)
  arc A21 (246.38, -132.8238) -> (246.752, -133.7219) centre (247.65, -132.8238) ccw
  line L25 (246.38, -132.8238) -> (246.38, -113.556)
  arc A22 (246.752, -112.658) -> (246.38, -113.556) centre (247.65, -113.556) ccw
  line L26 (246.752, -112.658) -> (249.292, -110.118)
  arc A23 (251.088, -110.118) -> (249.292, -110.118) centre (250.19, -111.0161) ccw
  line L27 (251.088, -110.118) -> (253.628, -112.658)
  arc A24 (273.422, -134.992) -> (272.5239, -134.62) centre (272.5239, -135.89) ccw
  line L28 (273.422, -134.992) -> (275.962, -137.532)
  arc A25 (275.962, -139.328) -> (275.962, -137.532) centre (275.0639, -138.43) ccw
  line L29 (275.962, -139.328) -> (273.422, -141.868)
  arc A26 (272.5239, -142.24) -> (273.422, -141.868) centre (272.5239, -140.97) ccw
  line L30 (272.5239, -142.24) -> (255.796, -142.24)
  arc A27 (254.898, -141.868) -> (255.796, -142.24) centre (255.796, -140.97) ccw
  line L31 (254.898, -141.868) -> (252.358, -139.328)
  arc A28 (252.358, -137.532) -> (252.358, -139.328) centre (253.256, -138.43) ccw
  line L32 (252.358, -137.532) -> (254.898, -134.992)
  arc A29 (255.796, -134.62) -> (254.898, -134.992) centre (255.796, -135.89) ccw
  line L33 (255.796, -134.62) -> (272.5239, -134.62)
  arc A30 (275.962, -169.808) -> (275.962, -168.012) centre (275.0639, -168.91) ccw
  line L34 (275.962, -169.808) -> (273.422, -172.348)
  arc A31 (272.5239, -172.72) -> (273.422, -172.348) centre (272.5239, -171.45) ccw
  line L35 (272.5239, -172.72) -> (255.796, -172.72)
  arc A32 (254.898, -172.348) -> (255.796, -172.72) centre (255.796, -171.45) ccw
  line L36 (254.898, -172.348) -> (252.358, -169.808)
  arc A33 (252.358, -168.012) -> (252.358, -169.808) centre (253.256, -168.91) ccw
  line L37 (252.358, -168.012) -> (254.898, -165.472)
  arc A34 (255.796, -165.1) -> (254.898, -165.472) centre (255.796, -166.37) ccw
  line L38 (255.796, -165.1) -> (272.5239, -165.1)
  arc A35 (273.422, -165.472) -> (272.5239, -165.1) centre (272.5239, -166.37) ccw
  line L39 (273.422, -165.472) -> (275.962, -168.012)
  arc A36 (277.232, -166.742) -> (279.028, -166.742) centre (278.13, -165.844) ccw
  line L40 (277.232, -166.742) -> (274.692, -164.202)
  arc A37 (274.32, -163.3039) -> (274.692, -164.202) centre (275.59, -163.3039) ccw
  line L41 (274.32, -163.3039) -> (274.32, -144.036)
  arc A38 (274.692, -143.138) -> (274.32, -144.036) centre (275.59, -144.036) ccw
  line L42 (274.692, -143.138) -> (277.232, -140.598)
  arc A39 (279.028, -140.598) -> (277.232, -140.598) centre (278.13, -141.496) ccw
  line L43 (279.028, -140.598) -> (281.568, -143.138)
  arc A40 (281.94, -144.036) -> (281.568, -143.138) centre (280.67, -144.036) ccw
  line L44 (281.94, -144.036) -> (281.94, -163.3039)
  arc A41 (281.568, -164.202) -> (281.94, -163.3039) centre (280.67, -163.3039) ccw
  line L45 (281.568, -164.202) -> (279.028, -166.742)
  arc A42 (192.668, -140.598) -> (190.872, -140.598) centre (191.77, -141.496) ccw
  line L46 (192.668, -140.598) -> (195.208, -143.138)
  arc A43 (195.58, -144.036) -> (195.208, -143.138) centre (194.31, -144.036) ccw
  line L47 (195.58, -144.036) -> (195.58, -163.3039)
  arc A44 (195.208, -164.202) -> (195.58, -163.3039) centre (194.31, -163.3039) ccw
  line L48 (195.208, -164.202) -> (192.668, -166.742)
  arc A45 (190.872, -166.742) -> (192.668, -166.742) centre (191.77, -165.844) ccw
  line L49 (190.872, -166.742) -> (188.332, -164.202)
  arc A46 (187.96, -163.3039) -> (188.332, -164.202) centre (189.23, -163.3039) ccw
  line L50 (187.96, -163.3039) -> (187.96, -144.036)
  arc A47 (188.332, -143.138) -> (187.96, -144.036) centre (189.23, -144.036) ccw
  line L51 (188.332, -143.138) -> (190.872, -140.598)
  arc A48 (254, -144.0361) -> (253.628, -143.1381) centre (252.73, -144.0361) ccw
  line L52 (254, -144.0361) -> (254, -163.3039)
  arc A49 (253.628, -164.202) -> (254, -163.3039) centre (252.73, -163.3039) ccw
  line L53 (253.628, -164.202) -> (251.088, -166.742)
  arc A50 (249.292, -166.742) -> (251.088, -166.742) centre (250.19, -165.8439) ccw
  line L54 (249.292, -166.742) -> (246.752, -164.202)
  arc A51 (246.38, -163.304) -> (246.752, -164.202) centre (247.65, -163.304) ccw
  line L55 (246.38, -163.304) -> (246.38, -144.0362)
  arc A52 (246.752, -143.1381) -> (246.38, -144.0362) centre (247.65, -144.0362) ccw
  line L56 (246.752, -143.1381) -> (249.292, -140.5981)
  arc A53 (251.0881, -140.5981) -> (249.292, -140.5981) centre (250.19, -141.4962) ccw
  line L57 (251.0881, -140.5981) -> (253.628, -143.1381)
  arc A54 (279.028, -110.118) -> (277.232, -110.118) centre (278.13, -111.016) ccw
  line L58 (279.028, -110.118) -> (281.568, -112.658)
  arc A55 (281.94, -113.5561) -> (281.568, -112.658) centre (280.67, -113.5561) ccw
  line L59 (281.94, -113.5561) -> (281.94, -132.824)
  arc A56 (281.568, -133.722) -> (281.94, -132.824) centre (280.67, -132.824) ccw
  line L60 (281.568, -133.722) -> (279.028, -136.262)
  arc A57 (277.232, -136.262) -> (279.028, -136.262) centre (278.13, -135.364) ccw
  line L61 (277.232, -136.262) -> (274.692, -133.722)
  arc A58 (274.32, -132.824) -> (274.692, -133.722) centre (275.59, -132.824) ccw
  line L62 (274.32, -132.824) -> (274.32, -113.5561)
  arc A59 (274.692, -112.658) -> (274.32, -113.5561) centre (275.59, -113.5561) ccw
  line L63 (274.692, -112.658) -> (277.232, -110.118)
  arc A60 (255.796, -104.14) -> (254.898, -104.512) centre (255.796, -105.41) ccw
  line L64 (255.796, -104.14) -> (272.5239, -104.14)
  arc A61 (273.422, -104.512) -> (272.5239, -104.14) centre (272.5239, -105.41) ccw
  line L65 (273.422, -104.512) -> (275.962, -107.052)
  arc A62 (275.962, -108.848) -> (275.962, -107.052) centre (275.0639, -107.95) ccw
  line L66 (275.962, -108.848) -> (273.422, -111.388)
  arc A63 (272.5239, -111.76) -> (273.422, -111.388) centre (272.5239, -110.49) ccw
  line L67 (272.5239, -111.76) -> (255.796, -111.76)
  arc A64 (254.898, -111.388) -> (255.796, -111.76) centre (255.796, -110.49) ccw
  line L68 (254.898, -111.388) -> (252.358, -108.848)
  arc A65 (252.358, -107.052) -> (252.358, -108.848) centre (253.256, -107.95) ccw
  line L69 (252.358, -107.052) -> (254.898, -104.512)
  arc A66 (223.148, -164.202) -> (223.52, -163.304) centre (222.25, -163.304) ccw
  line L70 (223.148, -164.202) -> (220.608, -166.742)
  arc A67 (218.812, -166.742) -> (220.608, -166.742) centre (219.71, -165.8439) ccw
  line L71 (218.812, -166.742) -> (216.272, -164.202)
  arc A68 (215.9, -163.3039) -> (216.272, -164.202) centre (217.17, -163.3039) ccw
  line L72 (215.9, -163.3039) -> (215.9, -144.0361)
  arc A69 (216.272, -143.1381) -> (215.9, -144.0361) centre (217.17, -144.0361) ccw
  line L73 (216.272, -143.1381) -> (218.8119, -140.5981)
  arc A70 (220.608, -140.5981) -> (218.8119, -140.5981) centre (219.71, -141.4962) ccw
  line L74 (220.608, -140.5981) -> (223.148, -143.1381)
  arc A71 (223.52, -144.0362) -> (223.148, -143.1381) centre (222.25, -144.0362) ccw
  line L75 (223.52, -144.0362) -> (223.52, -163.304)
  arc A72 (215.002, -104.512) -> (214.104, -104.14) centre (214.104, -105.41) ccw
  line L76 (215.002, -104.512) -> (217.542, -107.052)
  arc A73 (217.542, -108.848) -> (217.542, -107.052) centre (216.644, -107.95) ccw
  line L77 (217.542, -108.848) -> (215.002, -111.388)
  arc A74 (214.104, -111.76) -> (215.002, -111.388) centre (214.104, -110.49) ccw
  line L78 (214.104, -111.76) -> (197.3761, -111.76)
  arc A75 (196.478, -111.388) -> (197.3761, -111.76) centre (197.3761, -110.49) ccw
  line L79 (196.478, -111.388) -> (193.938, -108.848)
  arc A76 (193.938, -107.052) -> (193.938, -108.848) centre (194.8361, -107.95) ccw
  line L80 (193.938, -107.052) -> (196.478, -104.512)
  arc A77 (197.3761, -104.14) -> (196.478, -104.512) centre (197.3761, -105.41) ccw
  line L81 (197.3761, -104.14) -> (214.104, -104.14)
  arc A78 (192.668, -110.118) -> (190.872, -110.118) centre (191.77, -111.016) ccw
  line L82 (192.668, -110.118) -> (195.208, -112.658)
  arc A79 (195.58, -113.5561) -> (195.208, -112.658) centre (194.31, -113.5561) ccw
  line L83 (195.58, -113.5561) -> (195.58, -132.824)
  arc A80 (195.208, -133.722) -> (195.58, -132.824) centre (194.31, -132.824) ccw
  line L84 (195.208, -133.722) -> (192.668, -136.262)
  arc A81 (190.872, -136.262) -> (192.668, -136.262) centre (191.77, -135.364) ccw
  line L85 (190.872, -136.262) -> (188.332, -133.722)
  arc A82 (187.96, -132.824) -> (188.332, -133.722) centre (189.23, -132.824) ccw
  line L86 (187.96, -132.824) -> (187.96, -113.5561)
  arc A83 (188.332, -112.658) -> (187.96, -113.5561) centre (189.23, -113.5561) ccw
  line L87 (188.332, -112.658) -> (190.872, -110.118)
  circle A84 centre (234.95, -107.95) radius 3.175
  line L88 (272.5239, -171.958) -> (255.796, -171.958)
  line L89 (255.796, -165.862) -> (272.5239, -165.862)
  arc A85 (253.238, -144.0361) -> (247.142, -144.0361) centre (250.19, -144.0361) ccw
  line L90 (253.238, -144.0361) -> (253.238, -163.304)
  line L91 (247.142, -144.0361) -> (247.142, -163.304)
  arc A86 (247.142, -163.304) -> (253.238, -163.304) centre (250.19, -163.304) ccw
  arc A87 (255.796, -165.862) -> (255.796, -171.958) centre (255.796, -168.91) ccw
  arc A88 (272.5239, -171.958) -> (272.5239, -165.862) centre (272.5239, -168.91) ccw
  arc A89 (275.082, -163.304) -> (281.178, -163.304) centre (278.13, -163.304) ccw
  line L92 (275.082, -144.0361) -> (275.082, -163.304)
  arc A90 (281.178, -144.0361) -> (275.082, -144.0361) centre (278.13, -144.0361) ccw
  line L93 (281.178, -144.0361) -> (281.178, -163.304)
  line L94 (272.5239, -135.3821) -> (255.796, -135.3821)
  arc A91 (272.5239, -141.4781) -> (272.5239, -135.3821) centre (272.5239, -138.4301) ccw
  line L95 (255.796, -141.4781) -> (272.5239, -141.4781)
  arc A92 (255.796, -135.3821) -> (255.796, -141.4781) centre (255.796, -138.4301) ccw
  line L96 (272.5239, -104.9022) -> (255.796, -104.9022)
  arc A93 (272.5239, -110.9982) -> (272.5239, -104.9022) centre (272.5239, -107.9502) ccw
  line L97 (255.796, -110.9982) -> (272.5239, -110.9982)
  arc A94 (281.178, -113.5562) -> (275.082, -113.5562) centre (278.13, -113.5562) ccw
  line L98 (275.082, -132.8241) -> (275.082, -113.5562)
  line L99 (281.178, -132.824) -> (281.178, -113.5562)
  arc A95 (275.082, -132.8241) -> (281.178, -132.824) centre (278.13, -132.824) ccw
  arc A96 (255.796, -104.9022) -> (255.796, -110.9982) centre (255.796, -107.9502) ccw
  arc A97 (253.238, -113.5562) -> (247.142, -113.5562) centre (250.19, -113.5562) ccw
  line L100 (247.142, -132.8241) -> (247.142, -113.5562)
  line L101 (253.238, -132.8241) -> (253.238, -113.5562)
  arc A98 (247.142, -132.8241) -> (253.238, -132.8241) centre (250.19, -132.8241) ccw
  circle A99 centre (234.95, -107.95) radius 2.921
  line L102 (216.662, -144.0361) -> (216.662, -163.304)
  arc A100 (216.662, -163.304) -> (222.758, -163.304) centre (219.71, -163.304) ccw
  line L103 (222.758, -144.0361) -> (222.758, -163.304)
  arc A101 (222.758, -144.0361) -> (216.662, -144.0361) centre (219.71, -144.0361) ccw
  arc A102 (214.104, -141.4781) -> (214.104, -135.3821) centre (214.104, -138.4301) ccw
  line L104 (214.104, -141.4781) -> (197.3761, -141.4781)
  line L105 (197.3761, -135.3821) -> (214.104, -135.3821)
  arc A103 (197.3761, -135.3821) -> (197.3761, -141.4781) centre (197.3761, -138.4301) ccw
  arc A104 (194.818, -144.0361) -> (188.722, -144.0361) centre (191.77, -144.0361) ccw
  line L106 (188.722, -144.0361) -> (188.722, -163.304)
  line L107 (194.818, -144.0361) -> (194.818, -163.304)
  arc A105 (188.722, -163.304) -> (194.818, -163.304) centre (191.77, -163.304) ccw
  arc A106 (197.3761, -165.862) -> (197.3761, -171.958) centre (197.3761, -168.91) ccw
  line L108 (214.104, -165.862) -> (197.3761, -165.862)
  line L109 (197.3761, -171.958) -> (214.104, -171.958)
  arc A107 (214.104, -171.958) -> (214.104, -165.862) centre (214.104, -168.91) ccw
  line L110 (194.818, -132.8241) -> (194.818, -113.5562)
  line L111 (188.722, -132.824) -> (188.722, -113.5562)
  line L112 (214.104, -110.9982) -> (197.3761, -110.9982)
  line L113 (197.3761, -104.9022) -> (214.104, -104.9022)
  line L114 (216.662, -132.8241) -> (216.662, -113.5562)
  line L115 (222.758, -132.8241) -> (222.758, -113.5562)
  arc A108 (222.758, -113.5562) -> (216.662, -113.5562) centre (219.71, -113.5562) ccw
  arc A109 (214.104, -110.9982) -> (214.104, -104.9022) centre (214.104, -107.9502) ccw
  arc A110 (197.3761, -104.9022) -> (197.3761, -110.9982) centre (197.3761, -107.9502) ccw
  arc A111 (194.818, -113.5562) -> (188.722, -113.5562) centre (191.77, -113.5562) ccw
  arc A112 (216.662, -132.8241) -> (222.758, -132.8241) centre (219.71, -132.8241) ccw
  arc A113 (188.722, -132.824) -> (194.818, -132.8241) centre (191.77, -132.824) ccw
  dimension "d114" = 6.096
  dimension "d115" = 6.096
  dimension "d116" = 6.096
  dimension "d117" = 6.096
  dimension "d118" = 5.842
  constraint tangent L88 A87
  constraint tangent L89 A88
  constraint parallel L88 L89
  constraint tangent L90 A86
  constraint tangent L91 A86
  constraint parallel L90 L91
  constraint concentric A84 A99
  measures "d114" diameter of A88
  measures "d115" diameter of A87
  measures "d116" diameter of A85
  measures "d117" diameter of A86
  measures "d118" diameter of A99
extrude "Extrude21" add sketch "Sketch11" against normal blind 14.986 contours A0 L4 A1 L5 A2 L6 A3 L7 A4 L8 A5 L9 | A6 L10 A7 L11 A8 L12 A9 L13 A10 L14 A11 L15 | L16 A12 L17 A13 L18 A14 L19 A15 L20 A16 L21 A17 | A18 L22 A19 L23 A20 L24 A21 L25 A22 L26 A23 L27 | A24 L28 A25 L29 A26 L30 A27 L31 A28 L32 A29 L33 | A30 L34 A31 L35 A32 L36 A33 L37 A34 L38 A35 L39 | A36 L40 A37 L41 A38 L42 A39 L43 A40 L44 A41 L45 | A42 L46 A43 L47 A44 L48 A45 L49 A46 L50 A47 L51 | A48 L52 A49 L53 A50 L54 A51 L55 A52 L56 A53 L57 | A54 L58 A55 L59 A56 L60 A57 L61 A58 L62 A59 L63 | A60 L64 A61 L65 A62 L66 A63 L67 A64 L68 A65 L69 | A66 L70 A67 L71 A68 L72 A69 L73 A70 L74 A71 L75 | A72 L76 A73 L77 A74 L78 A75 L79 A76 L80 A77 L81 | A78 L82 A79 L83 A80 L84 A81 L85 A82 L86 A83 L87 | A84 bodies 1 2